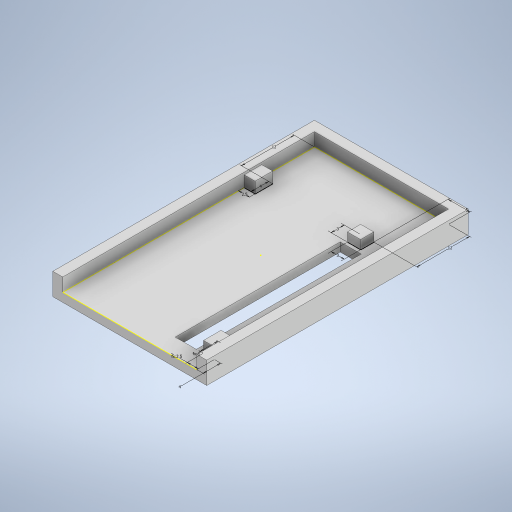
# Autodesk Inventor part: CROC Gluing Form V1
Saved by Autodesk Inventor 2024 (Build 280153000, 153)
## iProperties
Created: 2023-08-14
Part Number: CROC Gluing Form V1
Material: Generic
Document SubType Name: Modeling
Designer: cfang
Density: 1 g/cm^3
Appearance: Default
Author: cfang
Autodesk Inventor part; units mm, degrees
ref_plane "YZ Plane" through (0, 0, 0) normal (1, 0, 0) x (0, 1, 0)
ref_plane "XZ Plane" through (0, 0, 0) normal (0, 1, 0) x (-1, 0, 0)
ref_plane "XY Plane" through (0, 0, 0) normal (0, 0, 1) x (1, 0, 0)
sketch "Sketch1" plane through (0, 0, 0) normal (0, 1, 0) x (-1, 0, 0)
  line L0 (-17.5, -29.75) -> (17.5, -29.75)
  line L1 (17.5, -29.75) -> (17.5, 29.75)
  line L2 (17.5, 29.75) -> (-17.5, 29.75)
  line L3 (-17.5, 29.75) -> (-17.5, -29.75)
  line L4 (-17.5, -29.75) -> (17.5, 29.75) construction
  line L5 (17.5, -29.75) -> (-17.5, 29.75) construction
  point P0 (0, 0)
  dimension "d0" = 59.5
  dimension "d1" = 35
  constraints: 12 end point, 2 midpoint, 2 parallel, 1 horizontal, 1 perpendicular
  measures "d0" distance of L0.end L1.end
  measures "d1" distance of L1.end L2.end
extrude "Extrusion1" add sketch "Sketch1" along normal blind 5
sketch "Sketch2" plane through (0, 5, 0) normal (0, 1, 0) x (1, 0, 0)
  line L0 (-17.5, -29.75) -> (17.5, -29.75) projected
  line L1 (15.25, -29.75) -> (-15.25, -29.75)
  line L2 (-15.25, -29.75) -> (-15.25, 27.5)
  line L3 (-15.25, 27.5) -> (15.25, 27.5)
  line L4 (15.25, 27.5) -> (15.25, -29.75)
  line L5 (17.5, -29.75) -> (17.5, 29.75) projected
  line L6 (17.5, 29.75) -> (-17.5, 29.75) projected
  line L7 (-17.5, 29.75) -> (-17.5, -29.75) projected
  point P0 (0, 0)
  point P1 (-15.25, -29.75)
  dimension "d4" = 2.25
  dimension "d5" = 2.25
  dimension "d6" = 2.25
  constraints: 8 end point, 2 parallel, 1 horizontal, 1 perpendicular, 1 point on line
  measures "d4" distance between parallel lines of L5 L4
  measures "d5" distance between parallel lines of L6 L3
  measures "d6" distance between parallel lines of L7 L2
extrude "Extrusion2" cut sketch "Sketch2" against normal blind 3 contours L2 L3 L4 L0
sketch "Sketch3" plane through (0, 2, 0) normal (0, 1, 0) x (1, 0, 0)
  line L0 (10.25, 15.5) -> (7.25, 15.5)
  line L1 (7.25, 15.5) -> (7.25, 12.5)
  line L2 (7.25, 12.5) -> (10.25, 12.5)
  line L3 (10.25, 12.5) -> (10.25, 15.5)
  line L4 (-15.25, 27.5) -> (15.25, 27.5) projected
  line L5 (15.25, 27.5) -> (15.25, -29.75) projected
  line L6 (15.25, -25.75) -> (12.75, -25.75)
  line L7 (12.75, -25.75) -> (12.75, -21.75)
  line L8 (12.75, -21.75) -> (15.25, -21.75)
  line L9 (15.25, -21.75) -> (15.25, -25.75)
  line L10 (-15.25, -29.75) -> (-15.25, 27.5) projected
  line L11 (-15.25, 11.5) -> (-12.75, 11.5)
  line L12 (-12.75, 11.5) -> (-12.75, 15.5)
  line L13 (-12.75, 15.5) -> (-15.25, 15.5)
  line L14 (-15.25, 15.5) -> (-15.25, 11.5)
  line L15 (15.25, -29.75) -> (-15.25, -29.75) projected
  point P0 (0, 0)
  point P1 (15.25, -21.75)
  dimension "d9" = 3
  dimension "d10" = 3
  dimension "d21" = 12
  dimension "d22" = 5
  dimension "d23" = 2.5
  dimension "d24" = 4
  dimension "d25" = 4
  dimension "d26" = 2.5
  dimension "d27" = 12
  dimension "d28" = 4
  constraints: 24 end point, 6 parallel, 3 horizontal, 3 perpendicular, 2 point on line
  measures "d9" distance of L2.end L1.end
  measures "d10" distance of L1.end L0.end
  measures "d21" distance from line of L4 L0.start
  measures "d22" distance from line of L5 L0.start
  measures "d23" distance of L11.start L11.end
  measures "d24" distance of L11.end L12.end
  measures "d25" distance of L6.end L7.end
  measures "d26" distance of L6.start L6.end
  measures "d27" distance from line of L4 L12.end
  measures "d28" distance between parallel lines of L15 L6
extrude "Extrusion3" add sketch "Sketch3" along normal blind 2 contours L3 L2 L1 L0
extrude "Extrusion4" add sketch "Sketch3" along normal blind 2.5 contours L13 L12 L11 L10 | L5 L6 L7 L8
sketch "Sketch4" plane through (0, 2, 0) normal (0, 1, 0) x (1, 0, 0)
  line L0 (11.1804, 11.7081) -> (6.3882, 11.7081)
  line L1 (6.3882, 11.7081) -> (6.3882, -25.8012)
  line L2 (6.3882, -25.8012) -> (11.1804, -25.8012)
  line L3 (11.1804, -25.8012) -> (11.1804, 11.7081)
  point P0 (0, 0)
  constraints: 8 end point, 2 parallel, 1 horizontal, 1 perpendicular
extrude "Extrusion5" cut sketch "Sketch4" against normal through all
equation "\"d5\" = d4"
equation "\"d6\" = d4"
equation "\"d25\" = d24"
equation "\"d26\" = d23"
body "Solid1"
